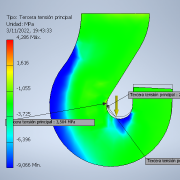
# Autodesk Inventor part: TAREA1
Saved by Autodesk Inventor 2020.5 (Build 245400000, 400)
## iProperties
Created: 2022-11-03
Part Number: TAREA1
Material: Acero, carbono AISI 1045
Document SubType Name: Modeling
Designer: André Aguirre Apolo
Density: 7.87 g/cm^3
Appearance: Semipulido
Mass: 791.333 g
Surface Area: 163.541 cm^2
Volume: 100.551 cm^3
Author: André Aguirre Apolo
Autodesk Inventor part; units mm, degrees
ref_plane "YZ Plane" through (0, 0, 0) normal (1, 0, 0) x (0, 1, 0)
ref_plane "XZ Plane" through (0, 0, 0) normal (0, 1, 0) x (-1, 0, 0)
ref_plane "XY Plane" through (0, 0, 0) normal (0, 0, 1) x (1, 0, 0)
sketch "Boceto1" plane through (0, 0, 0) normal (0, 0, 1) x (1, 0, 0)
  arc A0 (32.6864, 30.5882) -> (-30, 52) centre (5, 52) ccw
  line L0 (0, -19.2869) -> (0, 115.7212) projected
  line L1 (-80.1926, 0) -> (97.6435, 0) projected
  line L2 (0, 52) -> (-54.7874, 52) construction
  arc A1 (32.6864, 30.5882) -> (22.2384, 0) centre (72.2384, 0) ccw
  arc A2 (6.3623, 48.0288) -> (-7.5, 52) centre (0, 52) ccw
  arc A3 (-11.3876, 19.5913) -> (-17, 0) centre (20, 0) ccw
  line L3 (-10.0517, 21.7316) -> (6.3623, 48.0288)
  line L4 (-17, 0) -> (22.2384, 0)
  line L5 (-30, 52) -> (-30, 40.5821)
  line L6 (-30, 40.5821) -> (-7.5, 40.5821)
  line L7 (-7.5, 40.5821) -> (-7.5, 52)
  line L8 (-11.3876, 19.5913) -> (-10.0517, 21.7316)
  point P0 (0, 0)
  dimension "d0" = 70
  dimension "d1" = 52
  dimension "d2" = 5
  dimension "d3" = 52
  dimension "d4" = 100
  dimension "d5" = 15
  dimension "d7" = 17
  dimension "d8" = 10.0517
  dimension "d9" = 54.7874
  dimension "d10" = 40.5821
  dimension "d11" = 52
  dimension "d14" = 37
  dimension "d15" = 10
  dimension "d16" = 52
  constraints: 14 end point, 8 point on circle, 8 point on line, 4 centre point, 4 tangent, 2 perpendicular, 1 coincident, 1 collinear, 1 horizontal, 1 vertical
  measures "d0" diameter of A0
  measures "d1" distance from line of L1 A0.centre
  measures "d2" distance from line of L0 A0.centre
  measures "d3" distance between parallel lines of L1 L2
  measures "d4" diameter of A1
  measures "d5" diameter of A2
  measures "d7" distance of point (0, 0) L4.start
  measures "d8" distance from line of L3.start L0
  measures "d9" distance from line of L2.end L0
  measures "d10" distance between parallel lines of L6 L1
  measures "d11" distance from line of L7.end L1
  measures "d14" radius of A3
  measures "d16" distance from line of point (-7.5, 52) L1
extrude "Extrusión2" add sketch "Boceto1" along normal mid plane 40 contours A1 L1 L0 L3 A2 A0 | L0 A2 L7 L6 L5 A0 | L1 A3 L8 L3 L0
